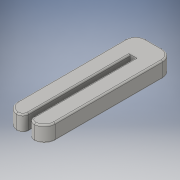
# Autodesk Inventor part: BaseClip
Saved by Autodesk Inventor 2016 (Build 200138000, 138)
## iProperties
Created: 2016-03-05
Part Number: BaseClip
Material: Generic
Document SubType Name: Modeling
Designer: yash
Density: 1 g/cm^3
Appearance: Default
Author: yash
Autodesk Inventor part; units mm, degrees
ref_plane "YZ Plane" through (0, 0, 0) normal (1, 0, 0) x (0, 1, 0)
ref_plane "XZ Plane" through (0, 0, 0) normal (0, 1, 0) x (-1, 0, 0)
ref_plane "XY Plane" through (0, 0, 0) normal (0, 0, 1) x (1, 0, 0)
sketch "Sketch1" plane through (0, 0, 0) normal (0, 1, 0) x (-1, 0, 0)
  line L0 (0, 0) -> (-4.7625, 0)
  line L1 (-4.7625, 0) -> (-4.7625, -31.75)
  line L2 (0, -1.7454) -> (0, 0)
  line L3 (-4.7625, -31.75) -> (-6.35, -31.75)
  line L4 (-11.1125, -1.7454) -> (-11.1125, -38.1)
  line L5 (-11.1125, -38.1) -> (0, -38.1)
  line L6 (0, -38.1) -> (0, -1.7454)
  line L7 (-6.35, -31.75) -> (-6.35, 0)
  line L8 (-6.35, 0) -> (-11.1125, 0)
  line L9 (-11.1125, 0) -> (-11.1125, -1.7454)
  dimension "d11" = 1.5875
  dimension "d12" = 38.1
  dimension "d13" = 6.35
  dimension "d14" = 4.7625
  constraints: 20 end point, 4 parallel, 3 equal length, 2 horizontal, 2 perpendicular
  measures "d11" distance of L1.end L3.end
  measures "d12" distance between parallel lines of L8 L5
  measures "d13" distance between parallel lines of L5 L3
  measures "d14" distance between parallel lines of L4 L7
extrude "Extrusion1" add sketch "Sketch1" along normal blind 4.7625
fillet "Fillet1" radius 3.175 4 edges at (0, 2.3813, -38.1) (11.1125, 2.3813, -38.1) (0, 2.3813, 0) (11.1125, 2.3813, 0)
fillet "Fillet2" radius 1.7272 2 edges at (6.35, 2.3813, 0) (4.7625, 2.3813, 0)
fillet "Fillet3" radius 0.4318 22 edges at (10.1826, 4.7625, -37.1701) (5.5563, 4.7625, -38.1) (0.9299, 4.7625, -37.1701) (0, 4.7625, -19.05) (0.8169, 4.7625, -1.0489) (4.1962, 4.7625, -0.4551) (4.7625, 4.7625, -16.742) (10.2956, 4.7625, -1.0489) (6.9163, 4.7625, -0.4551) (6.35, 4.7625, -16.742) (11.1125, 4.7625, -19.05) (10.1826, 0, -37.1701) (5.5563, 0, -38.1) (0.9299, 0, -37.1701) (0, 0, -19.05) (0.8169, 0, -1.0489) (4.1962, 0, -0.4551) (4.7625, 0, -16.742) (10.2956, 0, -1.0489) (6.9163, 0, -0.4551) (6.35, 0, -16.742) (11.1125, 0, -19.05)
body "Solid1"
